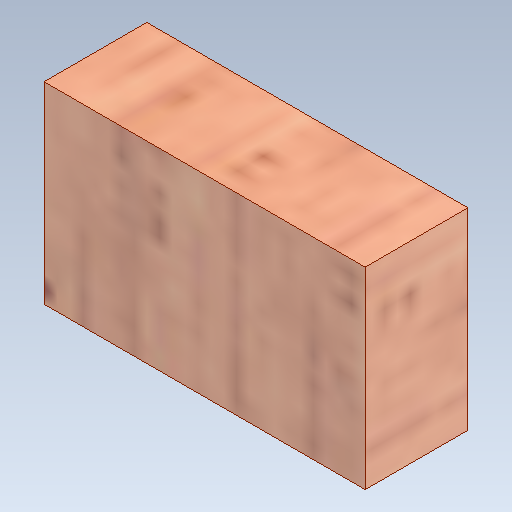
# Autodesk Inventor part: 0005-10-029 Activator Senzor Z
Saved by Autodesk Inventor 2020 (Build 240168000, 168)
## iProperties
Created: 2021-01-19
Part Number: 0005-10-029 Activator Senzor Z
Material: Generic
Document SubType Name: Modeling
Designer: Iulian Bors
Density: 1 g/cm^3
Appearance: White Oak - Natural Medium Gloss
Author: Iulian Bors
Subject: 029
Autodesk Inventor part; units mm, degrees
ref_plane "YZ Plane" through (0, 0, 0) normal (1, 0, 0) x (0, 1, 0)
ref_plane "XZ Plane" through (0, 0, 0) normal (0, 1, 0) x (-1, 0, 0)
ref_plane "XY Plane" through (0, 0, 0) normal (0, 0, 1) x (1, 0, 0)
sketch "Sketch1" plane through (0, 0, 0) normal (0, 0, 1) x (1, 0, 0)
  line L0 (-12.5, 7.5) -> (12.5, 7.5)
  line L1 (12.5, 7.5) -> (12.5, -7.5)
  line L2 (12.5, -7.5) -> (-12.5, -7.5)
  line L3 (-12.5, -7.5) -> (-12.5, 7.5)
  point P0 (0, 0)
  point P1 (-12.5, 0)
  point P2 (0, 7.5)
  dimension "d0" = 15
  dimension "d1" = 25
  constraints: 8 end point, 2 midpoint, 2 parallel, 1 horizontal, 1 horizontal alignment, 1 perpendicular, 1 vertical alignment
  measures "d0" distance of L2.end L0.start
  measures "d1" distance of L0.start L0.end
extrude "Extrusion1" add sketch "Sketch1" along normal blind 8
body "Solid1"
